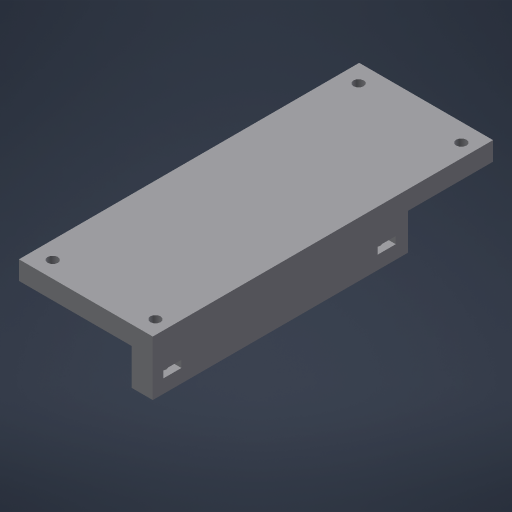
# Autodesk Inventor part: PCB BRACE
Saved by Autodesk Inventor 2023.3 (Build 273359000, 359)
## iProperties
RuleStatus: InUse
AfterDocSave0: file://Part Number Cleaner
Created: 2021-11-16
Material: Generic
Catalog Web Link: https://www.janelia.org/
Vendor: HHMI: JRC - jET
Document SubType Name: Modeling
Designer: goulett
Density: 1 g/cm^3
Appearance: Default
Part Number: PCB BRACE
LAB/DEPT: A. LEE (LAB)
DESIGN DEPARTMENT: HHMI: JRC - jET
ALTERED ITEM PART NUMBER: N/A
ALTERED ITEM VENDOR: N/A
ALTERED ITEM DESCRIPTION: N/A
Title: Standard
Author: goulett
Revision Number: 0
Autodesk Inventor part; units mm, degrees
ref_plane "YZ Plane" through (0, 0, 0) normal (1, 0, 0) x (0, 1, 0)
ref_plane "XZ Plane" through (0, 0, 0) normal (0, 1, 0) x (-1, 0, 0)
sketch "Sketch1" plane through (0, 0, 0) normal (0, 0, 1) x (1, 0, 0)
  line L0 (0, 0) -> (-4.7625, 0)
  line L1 (-4.7625, 0) -> (-4.7625, 17.646)
  line L2 (0, 17.646) -> (0, 0)
  line L3 (-20.447, 21.837) -> (9.525, 21.837)
  line L4 (9.525, 21.837) -> (9.525, 17.646)
  line L5 (-20.447, 17.646) -> (-20.447, 21.837)
  line L6 (9.525, 17.646) -> (0, 17.646)
  line L7 (-4.7625, 17.646) -> (-20.447, 17.646)
  point P0 (-2.3813, 0)
  dimension "d3" = 4.7625
  dimension "d4" = 4.191
  dimension "d5" = 29.972
  dimension "d6" = 21.837
  dimension "d8" = 9.525
  constraints: 16 end point, 4 parallel, 2 horizontal, 2 perpendicular, 1 collinear, 1 midpoint
  measures "d3" distance between parallel lines of L2 L1
  measures "d4" distance between parallel lines of L3 L6
  measures "d5" distance between parallel lines of L5 L4
  measures "d6" distance between parallel lines of L0 L3
  measures "d8" distance between parallel lines of L4 L2
extrude "Extrusion1" add sketch "Sketch1" along normal blind 76.2
sketch "Sketch2" plane through (-4.7625, 0, 0) normal (0, -1, 0) x (1, 0, 0)
  line L0 (0, 0) -> (4.7625, 0) projected
  line L1 (4.7625, 0) -> (4.7625, 76.2) projected
  line L2 (0, 76.2) -> (4.7625, 76.2) projected
  line L3 (0, 0) -> (0, 76.2) projected
  line L4 (0, 76.2) -> (4.7625, 76.2) projected
  circle A0 centre (2.2225, 62.2875) radius 2.2
  circle A1 centre (2.2225, 14.2875) radius 2.2
  circle A2 centre (2.2225, 14.2875) radius 1.143
  circle A3 centre (2.2225, 62.2875) radius 1.143
  point P0 (2.3813, 76.2)
  dimension "d52" = 2.286
  dimension "d53" = 2.286
  constraints: 4 centre point, 2 coincident, 1 midpoint, 4 other
  measures "d52" diameter of A2
  measures "d53" diameter of A3
chamfer "Chamfer1" distance 3.175 angle 45 2 edges at (-4.7625, 17.646, 38.1) (0, 17.646, 38.1)
extrude "Extrusion2" cut sketch "Sketch2" against normal blind 6.35 contours A2 | A3
ref_plane "Work Plane1" through (-4.7625, 3.81, 0) normal (0, -1, 0) x (1, 0, 0)
sketch "Sketch3" plane through (-4.7625, 3.81, 0) normal (0, -1, 0) x (1, 0, 0)
  circle A0 centre (2.2225, 62.2875) radius 1.016
  line L0 (4.7625, 60.2555) -> (1.0493, 60.2555)
  line L1 (1.0493, 60.2555) -> (-0.1239, 62.2875)
  line L2 (-0.1239, 62.2875) -> (1.0493, 64.3195)
  line L3 (1.0493, 64.3195) -> (4.7625, 64.3195)
  circle A1 centre (2.2225, 14.2875) radius 1.016
  line L4 (4.7625, 12.2555) -> (1.0493, 12.2555)
  line L5 (1.0493, 12.2555) -> (-0.1239, 14.2875)
  line L6 (-0.1239, 14.2875) -> (1.0493, 16.3195)
  line L7 (1.0493, 16.3195) -> (4.7625, 16.3195)
  line L8 (4.7625, 76.2) -> (4.7625, 0) projected
  circle A2 centre (2.2225, 14.2875) radius 1.143 projected
  circle A3 centre (2.2225, 62.2875) radius 1.143 projected
  dimension "d21" = 4.064
  dimension "d22" = 4.064
  constraints: 16 end point, 4 point on line, 2 centre point, 2 coincident, 2 concentric, 12 other
  measures "d21" distance between parallel lines of L4 L7
  measures "d22" distance between parallel lines of L3 L0
extrude "Extrusion3" cut sketch "Sketch3" against normal mid plane 1.5875 contours L0 L1 L2 L3 L8 | L8 L4 L5 L6 L7 | A1 | A2 | A3
sketch "Sketch5" plane through (-20.447, 17.646, 0) normal (0, -1, 0) x (1, 0, 0)
  circle A0 centre (3.907, 72.5295) radius 1 projected
  circle A1 centre (26.907, 72.5295) radius 1 projected
  circle A2 centre (26.907, 4.0455) radius 1 projected
  circle A3 centre (3.907, 4.0455) radius 1 projected
  point P0 (20.447, 0)
  constraints: 4 coincident
hole "Hole1" at (-16.54, 17.646, 72.5295) at (6.46, 17.646, 72.5295) at (6.46, 17.646, 4.0455) at (-16.54, 17.646, 4.0455) direction (0, 1, 0) diameter 2.286 depth 25.4 tip angle 118 counterbore diameter 4.064 counterbore depth 1.524
sketch "Sketch6" plane through (0, 0, 76.2) normal (0, 0, 1) x (1, 0, 0)
  line L0 (3.175, 17.646) -> (9.525, 17.646) projected
  line L1 (9.525, 17.646) -> (9.525, 21.837) projected
  line L2 (9.525, 21.837) -> (-20.447, 21.837) projected
  line L3 (-20.447, 21.837) -> (-20.447, 17.646) projected
  line L4 (-20.447, 17.646) -> (-7.9375, 17.646) projected
  line L5 (-4.7625, 14.471) -> (-7.9375, 17.646) projected
  line L6 (-4.7625, 14.471) -> (-4.7625, 0) projected
  line L7 (-4.7625, 0) -> (0, 0) projected
  line L8 (0, 0) -> (0, 14.471) projected
  line L9 (3.175, 17.646) -> (0, 14.471) projected
  line L10 (3.175, 17.646) -> (9.525, 17.646) projected
  line L11 (-7.9375, 17.646) -> (3.175, 17.646)
  constraints: 2 end point, 1 horizontal
extrude "Extrusion5" cut sketch "Sketch6" against normal blind 9.525 contours L9 L8 L7 L6 L5 L11
sketch "Sketch7" plane through (0, 0, 0) normal (0, 0, -1) x (-1, 0, 0)
  line L0 (0, 14.471) -> (-3.175, 17.646) projected
  line L1 (0, 0) -> (0, 14.471) projected
  line L2 (4.7625, 0) -> (0, 0) projected
  line L3 (4.7625, 14.471) -> (4.7625, 0) projected
  line L4 (7.9375, 17.646) -> (4.7625, 14.471) projected
  line L5 (20.447, 17.646) -> (7.9375, 17.646) projected
  line L6 (20.447, 21.837) -> (20.447, 17.646) projected
  line L7 (-9.525, 21.837) -> (20.447, 21.837) projected
  line L8 (-9.525, 17.646) -> (-9.525, 21.837) projected
  line L9 (-3.175, 17.646) -> (-9.525, 17.646) projected
  line L10 (-3.175, 17.646) -> (8.255, 17.646)
  line L11 (20.447, 17.646) -> (-9.525, 17.646) projected
  constraints: 2 end point, 1 collinear
extrude "Extrusion6" cut sketch "Sketch7" against normal blind 9.525 contours L0 L10 L4 L3 L2 L1
chamfer "Chamfer2" distance 3.175 angle 45 2 edges at (-2.3813, 17.646, 9.525) (-2.3813, 17.646, 66.675)
body "Solid1"
